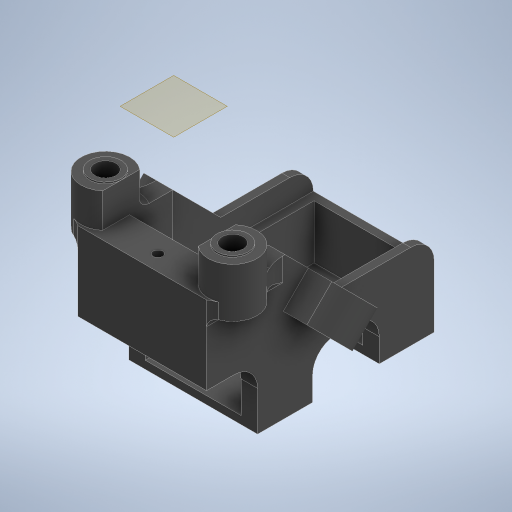
# Autodesk Inventor part: motor_cover_upper
Saved by Autodesk Inventor 2024.1 (Build 281209000, 209)
## iProperties
Created: 2024-12-19
Part Number: motor_cover_upper
Material: 一般
Document SubType Name: Modeling
Designer: hibik
Density: 1 g/cm^3
Appearance: 既定
Author: hibik
Autodesk Inventor part; units mm, degrees
ref_plane "YZ Plane" through (0, 0, 0) normal (1, 0, 0) x (0, 1, 0)
sketch "スケッチ1" plane through (0, 0, 0) normal (0, 1, 0) x (-1, 0, 0)
  line L0 (6.1, -5.5) -> (-6.1, -5.5)
  line L1 (-6.1, -5.5) -> (-6.1, 0)
  line L2 (-6.1, 0) -> (6.1, 0)
  line L3 (6.1, 0) -> (6.1, -5.5)
  line L4 (7.1, -5.5) -> (-7.1, -5.5)
  line L5 (-7.1, -5.5) -> (-7.1, 1)
  line L6 (-7.1, 1) -> (7.1, 1)
  line L7 (7.1, 1) -> (7.1, -5.5)
  point P0 (0, 0)
  point P1 (0, 0)
  point P2 (0, 1)
  point P3 (6.1, -5.5)
  point P4 (-6.1, -5.5)
  dimension "d0" = 12.2
  dimension "d1" = 5.5
  dimension "d2" = 14.2
  dimension "d3" = 1
  constraints: 16 end point, 4 parallel, 3 midpoint, 2 horizontal, 2 perpendicular, 1 coincident, 1 collinear, 1 vertical alignment
  measures "d0" distance of L1.end L2.end
  measures "d1" distance of L0.end L1.end
  measures "d2" distance of L5.end L6.end
  measures "d3" distance between parallel lines of L6 L2
extrude "押し出し1" add sketch "スケッチ1" along normal blind 17.05 contours L3 L2 L1 L4 L5 L6 L7
sketch "スケッチ2" plane through (0, 0, 0) normal (0, -1, 0) x (1, 0, 0)
  line L0 (7.1, -5.5) -> (6.1, -5.5) projected
  line L1 (-7.1, -5.5) -> (-7.1, 1) projected
  line L2 (7.1, -5.5) -> (-7.1, -5.5)
  line L3 (-7.1, -5.5) -> (-7.1, 1)
  line L4 (-7.1, 1) -> (7.1, 1)
  line L5 (7.1, 1) -> (7.1, -5.5)
  point P0 (0, 0)
  constraints: 8 end point, 2 parallel, 1 horizontal, 1 perpendicular
extrude "押し出し2" add sketch "スケッチ2" along normal blind 1
sketch "スケッチ7" plane through (-7.1, 17.05, -5.5) normal (-1, 0, 0) x (0, 0, 1)
  line L0 (6.5, -18.05) -> (6.5, 0) projected
  line L1 (10, 0) -> (6.5, 0)
  line L2 (6.5, 0) -> (6.5, -10)
  line L3 (6.5, -10) -> (10, -10)
  line L4 (10, -10) -> (10, 0)
  line L5 (10, 1.6) -> (10, 0) projected
  point P0 (5.5, -17.05)
  dimension "d26" = 10
  constraints: 8 end point, 2 parallel, 1 collinear, 1 horizontal, 1 perpendicular, 1 point on line
  measures "d26" distance of L1.start L3.end
extrude "押し出し7" add sketch "スケッチ7" against normal up to surface (14.2 mm away)
sketch "スケッチ9" plane through (-7.1, -1, -5.5) normal (-1, 0, 0) x (0, 0, 1)
  line L0 (6.5, 0) -> (6.5, 18.05) projected
  line L1 (6.5, 0) -> (0, 0) projected
  line L2 (6.5, 8.05) -> (3.5, 8.05)
  line L3 (3.5, 8.05) -> (3.5, 0)
  line L4 (3.5, 0) -> (6.5, 0)
  line L5 (6.5, 0) -> (6.5, 8.05)
  arc A0 (6.5, 8.05) -> (3.5, 5.05) centre (6.5, 5.05) ccw
  point P0 (5.5, 1)
  dimension "d31" = 3
  constraints: 8 end point, 2 parallel, 2 point on circle, 2 point on line, 2 tangent, 1 centre point, 1 horizontal, 1 perpendicular
  measures "d31" distance between parallel lines of L0 L3
extrude "押し出し9" cut sketch "スケッチ9" against normal through all contours L1 L3 A0 L0
ref_plane "作業平面2" through (-6.6, 19, -7.5) normal (0, -1, 0) x (-1, 0, 0)
sketch "スケッチ23" plane through (-6.1, 17.05, -5.5) normal (0, 0, -1) x (-1, 0, 0)
  line L0 (1, -18.05) -> (1, 0) projected
  line L1 (0, 0) -> (1, 0) projected
  line L2 (0, -17.05) -> (0, 0) projected
  line L3 (0, -17.05) -> (-12.2, -17.05) projected
  line L4 (-12.2, -17.05) -> (-12.2, 0) projected
  line L5 (-13.2, 0) -> (-12.2, 0) projected
  line L6 (-13.2, -18.05) -> (-13.2, 0) projected
  line L7 (1, -18.05) -> (-13.2, -18.05) projected
  line L8 (1, -10.2) -> (-13.2, -10.2)
  point P0 (-6.1, -17.05)
  point P1 (-12.2, -10.2)
  point P2 (0, -10.2)
  dimension "d84" = 10.2
  constraints: 2 end point, 2 point on line, 1 perpendicular
  measures "d84" distance between parallel lines of L5 L8
extrude "押し出し23" add sketch "スケッチ23" along normal blind 18 contours L7 L6 L8 L4 L3 L2 L0
sketch "スケッチ24" plane through (-6.1, 17.05, -23.5) normal (0, 0, -1) x (-1, 0, 0)
  line L0 (-13.2, -10.2) -> (-13.2, -18.05) projected
  line L1 (-13.2, -18.05) -> (1, -18.05)
  line L2 (1, -18.05) -> (1, -10.2)
  line L3 (1, -10.2) -> (-13.2, -10.2)
  line L4 (-13.2, -10.2) -> (-13.2, -18.05)
  point P0 (-6.1, -17.05)
  constraints: 8 end point, 2 parallel, 1 horizontal, 1 perpendicular
ref_plane "作業平面3" through (-7.1, 7.05, -28) normal (0, 0, -1) x (0, 1, 0)
extrude "押し出し24" add sketch "スケッチ24" along normal blind 1
sketch "スケッチ25" plane through (-7.1, 7.05, 4.5) normal (-1, 0, 0) x (0, 0, 1)
  line L0 (-6.5, -8.05) -> (-6.5, -3) projected
  arc A0 (-3.5, 0) -> (-6.5, -3) centre (-3.5, -3) ccw projected
  line L1 (-3.5, 0) -> (0, 0) projected
  line L2 (0, 0) -> (0, 10) projected
  line L3 (-10, 10) -> (0, 10) projected
  line L4 (-10, -0.2) -> (-10, 10) projected
  line L5 (-10, -0.2) -> (-29, -0.2) projected
  line L6 (-6.5, -8.05) -> (-29, -8.05) projected
  line L7 (-29, -8.05) -> (-29, -0.2) projected
  point P0 (-4.5, -7.05)
extrude "押し出し25" add sketch "スケッチ25" along normal blind 0.1
sketch "スケッチ26" plane through (-7.2, 7.05, 4.5) normal (-1, 0, 0) x (0, 0, 1)
  line L0 (-10, 10) -> (-4.5, 10) projected
  line L1 (-10, 10) -> (-20.2, -0.2)
  line L2 (-10, -0.2) -> (-10, 10) projected
  line L3 (-10, 2.8) -> (-29, 2.8)
  line L4 (-29, 2.8) -> (-29, -0.2)
  line L5 (-10, -0.2) -> (-29, -0.2) projected
  line L6 (-29, -8.05) -> (-6.5, -8.05) projected
  line L7 (-6.5, -8.05) -> (-6.5, -3) projected
  arc A0 (-3.5, 0) -> (-6.5, -3) centre (-3.5, -3) ccw projected
  line L8 (-3.5, 0) -> (0, 0) projected
  line L9 (0, 0) -> (0, 10) projected
  line L10 (0, 10) -> (-10, 10) projected
  line L11 (-10, 10) -> (-10, -0.2) projected
  line L12 (-10, -0.2) -> (-29, -0.2) projected
  line L13 (-29, -0.2) -> (-29, -8.05) projected
  line L14 (-29, -0.2) -> (-29, -8.05) projected
  point P0 (-4.5, -7.05)
  point P1 (-4.5, 10)
  point P2 (-17.2, 2.8)
  dimension "d91" = 45
  dimension "d92" = 3
  constraints: 6 end point, 3 point on line, 1 horizontal, 1 parallel, 1 perpendicular
  measures "d91" angle of L2 L1
  measures "d92" distance between parallel lines of L5 L3
extrude "押し出し26" add sketch "スケッチ26" along normal blind 1
mirror "ミラー5" about plane through (0, 0, 0) normal (1, 0, 0) of "押し出し25", "押し出し26"
sketch "スケッチ28" plane through (-7.2, 9.85, -12.7) normal (0, 0.7071068, -0.7071068) x (-1, 0, 0)
  line L0 (1, 0) -> (7, 0)
  line L1 (7, 0) -> (7, 6) construction
  line L2 (7, 6) -> (1, 6)
  line L3 (1, 6) -> (1, 0)
  circle A0 centre (4, 3) radius 3
  line L4 (1, 10.1823) -> (1, 0) projected
  circle A1 centre (4, 3) radius 1.6
  point P0 (-7.2, 2.0153)
  point P1 (4, 0)
  point P2 (4, 6)
  dimension "d99" = 6
  dimension "d100" = 3.2
  constraints: 8 end point, 4 tangent, 2 centre point, 2 parallel, 1 coincident, 1 horizontal, 1 perpendicular
  measures "d99" distance of L2.end L1.end
  measures "d100" diameter of A1
extrude "押し出し28" add sketch "スケッチ28" against normal blind 4.5
mirror "ミラー6" about plane through (0, 0, 0) normal (1, 0, 0) of "押し出し28"
sketch "スケッチ30" plane through (0, 17.05, 0) normal (0, 1, 0) x (1, 0, 0)
  circle A0 centre (0, -2.5) radius 0.85 construction
  circle A1 centre (0, -2.5) radius 0.6
  point P0 (0, 0)
  dimension "d105" = 1.2
  constraints: 1 centre point, 1 coincident
  measures "d105" diameter of A1
extrude "押し出し30" cut sketch "スケッチ30" against normal through all
ref_plane "作業平面4" through (-10.2, 22.1, -9.7183) normal (0, 1, 0) x (1, 0, 0)
sketch "スケッチ31" plane through (-10.2, 22.1, -9.7183) normal (0, 1, 0) x (1, 0, 0)
  circle A0 centre (0, 0) radius 1.35 construction
  circle A1 centre (10.2, -3.6183) radius 2.95 construction
  circle A2 centre (10.2, -3.6183) radius 10.8227 construction
  circle A3 centre (2.1, -10.7961) radius 3.1
  circle A4 centre (18.3, -10.7961) radius 3.1
  circle A5 centre (2.1, -10.7961) radius 1.35
  circle A6 centre (18.3, -10.7961) radius 1.35
  line L0 (4.1, -9.7183) -> (4.1, -4.2183) projected
  line L1 (16.3, -4.2183) -> (16.3, -9.7183) projected
  circle A7 centre (2.1, -10.7961) radius 2 construction
  line L2 (4.1, -9.7183) -> (4.1, -14.2183)
  line L3 (18.4, -14.2183) -> (2, -14.2183) projected
  line L4 (16.3, -9.7183) -> (4.1, -9.7183) projected
  line L5 (16.3, -9.7183) -> (16.3, -14.2183)
  line L6 (16.3, -9.7183) -> (16.3, -8.4276)
  point P0 (10.2, -9.7183)
  point P1 (16.3, -13.1647)
  point P2 (15.3934, -9.7183)
  point P3 (4.1, -13.1647)
  point P4 (4.1, -8.4276)
  dimension "d108" = 6.2
  dimension "d110" = 2.7
  dimension "d113" = 4
  constraints: 6 end point, 5 centre point, 4 coincident, 3 point on circle, 2 point on line, 2 vertical, 1 equal radius, 1 horizontal alignment, 1 tangent, 4 other
  measures "d108" diameter of A3
  measures "d110" diameter of A5
  measures "d113" diameter of A7
extrude "押し出し31" add sketch "スケッチ31" against normal blind 7 contours A3 L0 L2 | A4 L5 L1
fillet "フィレット5" radius 5 4 edges at (8.2, 16.075, 4.1763) (8.2, 16.075, -2.0205) (-8.2, 16.075, 4.1763) (-8.2, 16.075, -2.0205)
fillet "フィレット6" radius 1 6 edges at (-8.2, 15.1, -2.7417) (-8.2, 15.1, 3.4621) (8.2, 15.1, 3.4621) (8.2, 15.1, -2.7417) (8.0688, 17.05, -2.022) (-8.0688, 17.05, -2.022)
sketch "スケッチ32" plane through (-8.2, 7.05, 4.5) normal (-1, 0, 0) x (0, 0, 1)
  line L0 (-29, -8.05) -> (-6.5, -8.05) projected
  line L1 (-22, -8.05) -> (-13.5, -8.05)
  line L2 (-13.5, -8.05) -> (-13.5, -5.05)
  line L3 (-16.5, -2.05) -> (-19, -2.05)
  line L4 (-22, -5.05) -> (-22, -8.05)
  line L5 (-6.5, -8.05) -> (-6.5, -3) projected
  line L6 (-29, 2.8) -> (-29, -8.05) projected
  arc A0 (-19, -2.05) -> (-22, -5.05) centre (-19, -5.05) ccw
  arc A1 (-13.5, -5.05) -> (-16.5, -2.05) centre (-16.5, -5.05) ccw
  point P0 (-4.5, -7.05)
  point P1 (-22, -2.05)
  dimension "d116" = 7
  dimension "d117" = 7
  dimension "d118" = 6
  dimension "d119" = 3
  constraints: 8 end point, 4 point on circle, 4 tangent, 3 point on line, 2 centre point, 2 parallel, 1 equal radius, 1 horizontal, 1 perpendicular
  measures "d116" distance between parallel lines of L5 L2
  measures "d117" distance between parallel lines of L6 L4
  measures "d118" distance of point (-22, -2.05) L1.start
  measures "d119" radius of A0
extrude "押し出し32" cut sketch "スケッチ32" against normal through all
fillet "フィレット7" radius 3 2 edges at (-7.7, 9.85, -24.5) (7.7, 9.85, -24.5)
sketch "スケッチ33" plane through (-10.2, 22.1, -9.7183) normal (0, 1, 0) x (1, 0, 0)
  line L0 (2, -12.1424) -> (2, -14.2183) projected
  line L1 (4.1, -13.1647) -> (4.1, -8.4276) projected
  arc A0 (4.1, -8.4276) -> (4.1, -13.1647) centre (2.1, -10.7961) ccw projected
  circle A1 centre (2.1, -10.7961) radius 1.35 projected
  line L2 (18.4, -9.4498) -> (18.4, -4.5033) projected
  line L3 (16.3, -8.4276) -> (16.3, -13.1647) projected
  arc A2 (16.3, -13.1647) -> (16.3, -8.4276) centre (18.3, -10.7961) ccw projected
  circle A3 centre (18.3, -10.7961) radius 1.35 projected
  point P0 (10.2, -9.7183)
  point P1 (2, -7.6977)
  point P2 (2, -9.4498)
  point P3 (18.4, -7.6977)
  constraints: 1 other
extrude "押し出し33" cut sketch "スケッチ33" against normal blind 0.7
sketch "スケッチ34" plane through (-10.2, 21.4, -9.7183) normal (0, 1, 0) x (1, 0, 0)
  circle A0 centre (2.1, -10.7961) radius 1.35 projected
  circle A1 centre (18.3, -10.7961) radius 1.35 projected
  circle A2 centre (2.1, -10.7961) radius 2
  circle A3 centre (18.3, -10.7961) radius 2
  point P0 (10.2, -9.7183)
  dimension "d125" = 4
  dimension "d126" = 4
  constraints: 2 centre point, 2 coincident
  measures "d125" diameter of A2
  measures "d126" diameter of A3
extrude "押し出し34" add sketch "スケッチ34" along normal blind 0.2
equation "\"d117\" = d116"
